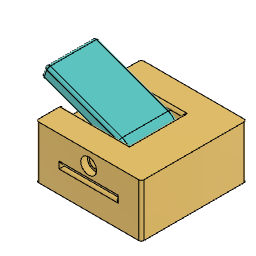
Anschlag_20x0.5MM (Autodesk Fusion 360 design; units mm, degrees)
Autodesk Fusion 360 part; units mm, degrees
sketch "Sketch1" plane through (0, 0, 0) normal (0, 1, 0) x (1, 0, 0)
  line L0 (0, 0) -> (40, 0)
  line L1 (40, 0) -> (40, -20)
  line L2 (40, -20) -> (0, -20)
  line L3 (0, -20) -> (0, 0)
  line L4 (9.75, -10) -> (30.25, -10)
  line L5 (30.25, -10) -> (30.25, -9.4)
  line L6 (30.25, -9.4) -> (9.75, -9.4)
  line L7 (9.75, -9.4) -> (9.75, -10)
  line L8 (0, -15) -> (14.5, -15)
  line L9 (14.5, -15) -> (14.5, -10)
  circle A0 centre (20, -15) radius 1.25
  line L10 (25.5, -10) -> (25.5, -20)
  circle A1 centre (20, -15) radius 3
  dimension "d1" = 40
  dimension "d2" = 20
  dimension "d3" = 0.6
  dimension "d5" = 20.5
  dimension "d6" = 9.75
  dimension "d22" = 10
  dimension "d41" = 0
  dimension "d42" = 0
  dimension "d43" = 0
  dimension "d44" = 0
  dimension "d62" = 11
  dimension "d63" = 14.5
  dimension "d64" = 2.5
  dimension "d69" = 5.5
  dimension "d70" = 6
  constraint horizontal L0
  constraint vertical L1
  constraint horizontal L2
  constraint vertical L3
  constraint coincident L0.start L3.end
  constraint horizontal L4
  constraint vertical L5
  constraint horizontal L6
  constraint vertical L7
  constraint coincident L3 L8.start
  constraint perpendicular L3 L8
  constraint coincident L4 L9.end
  constraint perpendicular L4 L9
  constraint coincident L2 L10.end
  constraint perpendicular L2 L10
  constraint horizontal L8.end A0.centre
  constraint concentric A0 A1
  measures "d1" distance of L0.start L0.end
  measures "d2" distance of L0.start L2.end
  measures "d3" distance of L4.end L5.end
  measures "d5" distance of L4.start L4.end
  measures "d6" distance of L1 L5.end
  measures "d22" distance of L2 L4
  measures "d62" distance of L9 L10
  measures "d63" distance of L8.start L8.end
  measures "d64" diameter of A0
  measures "d69" distance of A0.centre L10
  measures "d70" diameter of A1
extrude "Extrude1" add sketch "Sketch1" along normal blind 40 contours L0 L1 L2 L3 L4 L5 L6 L7 L8 L9 L10 | L2 L3 L4 L8 L9 L10 | A0 | A1 makes body 1
sketch "Sketch1 (2)" plane through (0, 0, 0) normal (0, 1, 0) x (1, 0, 0) in component "Component"
  line L0 (30.0688, -21.4416) -> (20.0688, -21.4416)
  line L1 (20.0688, -21.4416) -> (20.0688, -11.4416)
  line L2 (20.0688, -11.4416) -> (30.0688, -11.4416)
  line L3 (30.0688, -11.4416) -> (30.0688, -21.4416)
  circle A0 centre (25.0688, -16.4416) radius 1.25
  circle A1 centre (25.0688, -16.4416) radius 5
  line L4 (20.0688, -21.4416) -> (-4.9312, -21.4416)
  line L5 (-4.9312, -21.4416) -> (-4.9312, -16.4416)
  line L6 (-4.9312, -16.4416) -> (20.0688, -16.4416)
  line L7 (20.0688, -16.4416) -> (20.0688, -21.4416)
  arc A2 (30.0688, -15.8416) -> (20.0688, -15.8416) centre (25.0688, -15.8416) ccw
  dimension "d9" = 2.5
  dimension "d13" = 10
  dimension "d14" = 10
  dimension "d19" = 10
  dimension "d20" = 5
  dimension "d29" = 5
  dimension "d30" = 25
  dimension "d37" = 0
  dimension "d38" = 0
  dimension "d39" = 0
  dimension "d40" = 0
  dimension "d57" = 0.6
  dimension "d58" = 5
  dimension "d59" = 5
  constraint horizontal L0
  constraint vertical L1
  constraint horizontal L2
  constraint vertical L3
  constraint concentric A0 A1
  constraint horizontal L4
  constraint vertical L5
  constraint horizontal L6
  constraint vertical L7
  constraint coincident L3 A2.start
  constraint coincident L1 A2.end
  constraint horizontal A2.end A2.start
  measures "d9" diameter of A0
  measures "d13" distance of L1.end L2.end
  measures "d14" distance of L0.start L2.end
  measures "d19" diameter of A1
  measures "d20" distance of L3 A0.centre
  measures "d29" distance of L4.end L5.end
  measures "d30" distance of L0.end L4.end
  measures "d57" distance of L6.end A2.end
  measures "d58" radius of A2
  measures "d59" distance of L0 A0.centre
extrude "Extrude1'" add sketch "Sketch1 (2)" against normal blind 19.5 separate body contours L0 L1 A1 L7 | A1 | L2 L3 A1 A2 | L1 L4 L5 L6 L7 | L1 L2 A1 A2 | L2 A2 makes body 2 in component "Component"
extrude "Extrude2" cut sketch "Sketch1" along normal blind 20 and the other way blind -10 contours L4 L5 L6 L7 bodies 1
extrude "Extrude3" cut sketch "Sketch1" along normal blind 30 and the other way blind -10 contours L2 L3 L4 L8 L9 L10 | A0 | A1 bodies 1
extrude "Extrude4" cut sketch "Sketch1" along normal blind 44 contours A0 bodies 1
extrude "Extrude6" cut sketch "Sketch1" along normal blind 2.5 contours A1 bodies 1
fillet "Fillet1" radius 1 19 edges at (12.75, 30, 20) (12.75, 10, 20) (0, 0, 10) (0, 40, 10) (40, 0, 10) (40, 40, 10) (14.5, 20, 15) (25.5, 20, 10) (14.5, 20, 10) (25.5, 20, 20) (18.8346, 2.5, 14.548) (20, 0, 10) (20, 0, 9.4) (9.75, 0, 9.7) (30.25, 0, 9.7) (20, 40, 9.4) (20, 40, 10) (30.25, 40, 9.7) (9.75, 40, 9.7) on bodies 1
fillet "Fillet1'" radius 1 16 edges at (20.0688, 0, 16.1416) (25.0688, 0, 10.8416) (30.0688, 0, 16.1416) (28.6044, 0, 19.9771) (10.0688, 0, 21.4416) (7.5688, 0, 16.4416) (20.0688, -19.5, 16.1416) (25.0688, -19.5, 10.8416) (30.0688, -19.5, 16.1416) (28.6044, -19.5, 19.9771) (10.0688, -19.5, 21.4416) (7.5688, -19.5, 16.4416) (-4.9312, -19.5, 18.9416) (-4.9312, 0, 18.9416) (-4.9312, -9.75, 16.4416) (-4.9312, -9.75, 21.4416) on bodies 2 in component "Component"
sketch "Sketch2" plane through (0, 0, 9.4) normal (0, 0, 1) x (-1, 0, 0)
  line L0 (-30.25, -1) -> (-30.25, -39)
  line L1 (-9.75, -39) -> (-9.75, -1)
  circle A0 centre (-9, -35) radius 1.5
  circle A1 centre (-9, -5) radius 1.5
  line L2 (-30.25, -39) -> (-9.75, -39)
  line L3 (-9.75, -1) -> (-30.25, -1)
  dimension "d67" = 3
  dimension "d68" = 3
  measures "d67" diameter of A0
  measures "d68" diameter of A1
extrude "Extrude5" [suppressed]
component "Component" placed x (1, 0, 0) y (0, 1, 0) z (0, 0, 1) at (-5.0688, 29.5, -1.4416)
equation "d6 = ( d1 - d5 ) / 2"
equation "d63 = ( d1 - d62 ) / 2"
equation "d69 = d62 / 2"
